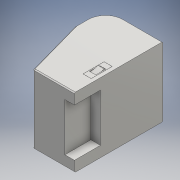
# Autodesk Inventor part: printer2
Saved by Autodesk Inventor 2016 (Build 200138000, 138)
## iProperties
Created: 2018-11-07
Part Number: printer2
Material: PPS Plastic
Document SubType Name: Modeling
Designer: hovm
Density: 1.637 g/cm^3
Appearance: Smooth - White
Author: hovm
Autodesk Inventor part; units mm, degrees
ref_plane "YZ Plane" through (0, 0, 0) normal (1, 0, 0) x (0, 1, 0)
ref_plane "XZ Plane" through (0, 0, 0) normal (0, 1, 0) x (-1, 0, 0)
ref_plane "XY Plane" through (0, 0, 0) normal (0, 0, 1) x (1, 0, 0)
sketch "Sketch1" plane through (0, 0, 0) normal (0, 0, 1) x (1, 0, 0)
  line L0 (-83.7217, 0) -> (0, 0)
  line L1 (0, 0) -> (0, 185)
  line L2 (0, 185) -> (-82, 185)
  line L3 (-120, 147) -> (-120, 122)
  line L4 (-120, 122) -> (-86.6116, 2.1946)
  arc A0 (-82, 185) -> (-120, 147) centre (-82, 147) ccw
  arc A1 (-86.6116, 2.1946) -> (-83.7217, 0) centre (-83.7217, 3) ccw
  point P0 (-86, 0)
  dimension "d0" = 185
  dimension "d1" = 86
  dimension "d2" = 122
  dimension "d3" = 120
  dimension "d4" = 38
  dimension "d5" = 3
  constraints: 10 end point, 4 point on circle, 4 tangent, 3 perpendicular, 2 centre point, 2 point on line, 1 horizontal
  measures "d0" distance of L0.end L1.end
  measures "d1" distance of point (-86, 0) L0.end
  measures "d2" vertical distance of L3.end point (-86, 0)
  measures "d3" distance between parallel lines of L1 L3
  measures "d4" radius of A0
  measures "d5" radius of A1
extrude "Extrusion1" add sketch "Sketch1" along normal mid plane 145
sketch "Sketch2" plane through (-86.6116, 2.1946, -72.5) normal (-0.9632913, -0.2684582, 0) x (0, 0, 1)
  line L0 (27.5, 42) -> (117.5, 42)
  line L1 (118.5, 43) -> (118.5, 91)
  line L2 (117.5, 92) -> (27.5, 92)
  line L3 (26.5, 91) -> (26.5, 43)
  line L4 (26.5, 42) -> (118.5, 92) construction
  line L5 (118.5, 42) -> (26.5, 92) construction
  line L6 (145, 0) -> (0, 0) projected
  arc A0 (27.5, 92) -> (26.5, 91) centre (27.5, 91) ccw
  arc A1 (26.5, 43) -> (27.5, 42) centre (27.5, 43) ccw
  arc A2 (117.5, 42) -> (118.5, 43) centre (117.5, 43) ccw
  arc A3 (118.5, 91) -> (117.5, 92) centre (117.5, 91) ccw
  point P0 (72.5, -25.3657)
  point P1 (72.5, 67)
  point P2 (72.5, 67)
  dimension "d8" = 50
  dimension "d9" = 92
  dimension "d10" = 42
  dimension "d11" = 1
  constraints: 12 end point, 8 point on circle, 8 point on line, 8 tangent, 4 centre point, 3 equal radius, 3 midpoint, 2 parallel, 1 horizontal, 1 perpendicular, 1 vertical alignment
  measures "d8" distance of L5.start L4.end
  measures "d9" distance of L4.end L5.end
  measures "d10" distance between parallel lines of L0 L6
  measures "d11" radius of A0
extrude "Extrusion2" add sketch "Sketch2" along normal blind 3
sketch "Sketch3" plane through (-89.5015, 1.3893, -72.5) normal (-0.9632913, -0.2684582, 0) x (0, 0, 1)
  line L0 (117.5, 92) -> (27.5, 92) projected
  arc A0 (27.5, 92) -> (26.5, 91) centre (27.5, 91) ccw projected
  line L1 (26.5, 91) -> (26.5, 43) projected
  arc A1 (26.5, 43) -> (27.5, 42) centre (27.5, 43) ccw projected
  line L2 (27.5, 42) -> (117.5, 42) projected
  arc A2 (117.5, 42) -> (118.5, 43) centre (117.5, 43) ccw projected
  line L3 (118.5, 43) -> (118.5, 91) projected
  arc A3 (118.5, 91) -> (117.5, 92) centre (117.5, 91) ccw projected
  line L4 (28.5, 90) -> (116.5, 90)
  line L5 (116.5, 90) -> (116.5, 44)
  line L6 (116.5, 44) -> (28.5, 44)
  line L7 (28.5, 44) -> (28.5, 90)
  point P0 (72.5, -25.3657)
  dimension "d14" = 2
  constraints: 8 end point, 3 other
  measures "d14" distance between parallel lines of L0 L4
extrude "Extrusion3" cut sketch "Sketch3" against normal blind 3 contours L4 L5 L6 L7
sketch "Sketch4" plane through (0, 0, 0) normal (0, 0, 1) x (1, 0, 0)
  line L0 (-98.4238, 44.5794) -> (-110.7729, 88.8908) projected
  line L1 (-110.7729, 88.8908) -> (-81.1902, 78.6338)
  line L2 (-80.5941, 78.6154) -> (-77.0419, 79.6053)
  line L3 (-101.3137, 43.7741) -> (-113.6627, 88.0855) projected
  line L4 (-77.0419, 79.6053) -> (-74.3573, 69.9724)
  line L5 (-74.3573, 69.9724) -> (-77.9095, 68.9825)
  line L6 (-78.4101, 68.6584) -> (-98.4238, 44.5794)
  arc A0 (-81.1902, 78.6338) -> (-80.5941, 78.6154) centre (-80.8626, 79.5787) ccw
  arc A1 (-77.9095, 68.9825) -> (-78.4101, 68.6584) centre (-77.6411, 68.0192) ccw
  point P0 (0, 0)
  point P1 (-80.895, 78.5315)
  point P2 (-78.2105, 68.8986)
  dimension "d17" = 10
  dimension "d18" = 30
  dimension "d19" = 18
  dimension "d20" = 4
  dimension "d21" = 4
  dimension "d22" = 1
  constraints: 10 end point, 4 point on circle, 4 point on line, 4 tangent, 3 perpendicular, 2 centre point, 1 equal radius
  measures "d17" distance of L2.end L4.end
  measures "d18" distance between parallel lines of L4 L0
  measures "d19" distance from line of L5 L0.start
  measures "d20" distance of L4.end point (-78.21, 68.899)
  measures "d21" distance of point (-80.895, 78.532) L2.end
  measures "d22" radius of A0
extrude "Extrusion4" cut sketch "Sketch4" along normal mid plane 88
chamfer "Chamfer1" distance 2 angle 45 12 edges at (-103.3058, 62.0973, 72.5) (-85.5361, 0.6108, 72.5) (-41.8609, 0, 72.5) (-120, 134.5, 72.5) (-108.8701, 173.8701, 72.5) (-41, 185, 72.5) (-103.3058, 62.0973, -72.5) (-85.5361, 0.6108, -72.5) (-41.8609, 0, -72.5) (-120, 134.5, -72.5) (-108.8701, 173.8701, -72.5) (-41, 185, -72.5)
sketch "Sketch5" plane through (0, 0, 72.5) normal (0, 0, 1) x (1, 0, 0)
  line L0 (-8, 43) -> (-25, 43)
  line L1 (-25, 43) -> (-25, 87)
  line L2 (-25, 87) -> (-8, 87)
  line L3 (-8, 87) -> (-8, 43)
  line L4 (-8, 43) -> (-25, 87) construction
  line L5 (-25, 43) -> (-8, 87) construction
  line L6 (-83.7217, 0) -> (0, 0) projected
  line L7 (0, 2) -> (0, 183) projected
  point P0 (-16.5, 65)
  dimension "d28" = 17
  dimension "d29" = 65
  dimension "d30" = 16.5
  dimension "d31" = 44
  constraints: 12 end point, 2 midpoint, 2 parallel, 1 horizontal, 1 perpendicular
  measures "d28" distance of L1.end L2.end
  measures "d29" distance from line of point (-16.5, 65) L6
  measures "d30" distance from line of L7 point (-16.5, 65)
  measures "d31" distance of L0.end L1.end
extrude "Extrusion5" cut sketch "Sketch5" against normal blind 0.1
sketch "Sketch6" plane through (0, 0, 72.4) normal (0, 0, 1) x (1, 0, 0)
  line L0 (-10, 55.5) -> (-23, 55.5)
  line L1 (-23, 55.5) -> (-23, 74.5)
  line L2 (-23, 74.5) -> (-10, 74.5)
  line L3 (-10, 74.5) -> (-10, 55.5)
  line L4 (-10, 55.5) -> (-23, 74.5) construction
  line L5 (-23, 55.5) -> (-10, 74.5) construction
  line L6 (-8, 87) -> (-8, 43) projected
  line L7 (-25, 87) -> (-8, 87) projected
  point P0 (0, 0)
  point P1 (-16.5, 65)
  point P2 (-16.5, 65)
  point P3 (-8, 65)
  point P4 (-16.5, 65)
  point P5 (-16.5, 87)
  dimension "d34" = 19
  dimension "d35" = 13
  constraints: 12 end point, 6 midpoint, 2 parallel, 1 horizontal, 1 horizontal alignment, 1 perpendicular, 1 vertical alignment
  measures "d34" distance of L0.end L1.end
  measures "d35" distance of L0.start L0.end
extrude "Extrusion6" cut sketch "Sketch6" against normal blind 2
chamfer "Chamfer2" distance 1 angle 45 2 edges at (-16.5, 74.5, 72.4) (-16.5, 55.5, 72.4)
sketch "Sketch7" plane through (-10, 55.5, 70.4) normal (-1, 0, 0) x (0, 0, 1)
  line L0 (2, 31.5) -> (2, -12.5) projected
  line L1 (2, 9.5) -> (-13.8786, 9.5) construction
  line L2 (2, 0) -> (-11.9991, 0) construction
  line L3 (-11.9991, 0) -> (-11.9991, 19) construction
  line L4 (-11.9991, 19) -> (2, 19) construction
  arc A0 (4.6177, 17.685) -> (0.2099, 0) centre (58.3508, -5.099) ccw
  arc A1 (4.6177, 17.685) -> (-0.8249, 19) centre (-0.8249, 7.0798) ccw
  line L5 (0.2099, 0) -> (-0.8249, 19)
  point P0 (-70.4, -55.5)
  dimension "d41" = 19
  constraints: 10 end point, 4 point on circle, 4 point on line, 2 centre point, 2 horizontal, 2 perpendicular, 1 midpoint, 1 tangent, 1 other
  measures "d41" distance of L2.end L3.end
extrude "Extrusion7" add sketch "Sketch7" along normal up to surface (13 mm away)
fillet "Fillet1" radius 1.5 1 edges at (-16.5, 73.185, 75.0177)
sketch "Sketch9" plane through (-83.7217, 0, -70.5) normal (0, -1, 0) x (1, 0, 0)
  line L0 (103.7217, 20.5) -> (63.7217, 20.5)
  line L1 (63.7217, 20.5) -> (63.7217, 120.5)
  line L2 (63.7217, 120.5) -> (103.7217, 120.5)
  line L3 (103.7217, 120.5) -> (103.7217, 20.5)
  line L4 (103.7217, 20.5) -> (63.7217, 120.5) construction
  line L5 (63.7217, 20.5) -> (103.7217, 120.5) construction
  point P0 (83.7217, 70.5)
  dimension "d45" = 40
  dimension "d46" = 100
  constraints: 12 end point, 2 midpoint, 2 parallel, 1 horizontal, 1 perpendicular
  measures "d45" distance of L1.end L2.end
  measures "d46" distance of L2.end L0.start
extrude "Extrusion8" cut sketch "Sketch9" against normal blind 54.25
equation "\"d21\" = d20"
body "Solid1"
